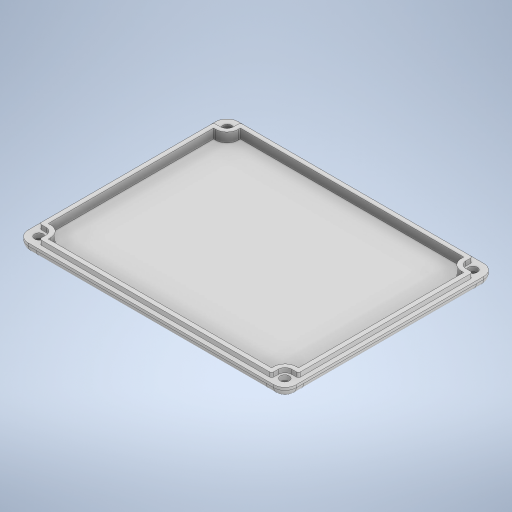
# Autodesk Inventor part: Couvercle_aluminium
Saved by Autodesk Inventor 2024 (Build 280153000, 153)
## iProperties
Created: 2024-08-30
Part Number: Couvercle_aluminium
Material: Générique
Document SubType Name: Modeling
Designer: malam
Density: 1 g/cm^3
Appearance: Par défaut
Author: malam
Autodesk Inventor part; units mm, degrees
ref_plane "YZ Plane" through (0, 0, 0) normal (1, 0, 0) x (0, 1, 0)
ref_plane "XZ Plane" through (0, 0, 0) normal (0, 1, 0) x (-1, 0, 0)
ref_plane "XY Plane" through (0, 0, 0) normal (0, 0, 1) x (1, 0, 0)
sketch "Esquisse1" plane through (0, 0, 0) normal (0, 1, 0) x (-1, 0, 0)
  arc A0 (55, -47) -> (60, -42) centre (55, -42) ccw
  line L0 (60, -42) -> (60, 42)
  arc A1 (60, 42) -> (55, 47) centre (55, 42) ccw
  line L1 (55, 47) -> (-55, 47)
  arc A2 (-55, 47) -> (-60, 42) centre (-55, 42) ccw
  line L2 (-60, 42) -> (-60, -42)
  arc A3 (-60, -42) -> (-55, -47) centre (-55, -42) ccw
  line L3 (-55, -47) -> (55, -47)
  circle A4 centre (55, 42.115) radius 2
  circle A5 centre (55, -42.115) radius 2
  circle A6 centre (-55, 42.115) radius 2
  circle A7 centre (-55, -42.115) radius 2
  arc A8 (55, -39) -> (52, -42) centre (55, -42) ccw
  line L4 (52, -42) -> (52, -44)
  arc A9 (51, -45) -> (52, -44) centre (51, -44) ccw
  line L5 (51, -45) -> (-51, -45)
  arc A10 (-52, -44) -> (-51, -45) centre (-51, -44) ccw
  line L6 (-52, -44) -> (-52, -42)
  arc A11 (-52, -42) -> (-55, -39) centre (-55, -42) ccw
  line L7 (-55, -39) -> (-57, -39)
  arc A12 (-58, -38) -> (-57, -39) centre (-57, -38) ccw
  line L8 (-58, -38) -> (-58, 38)
  arc A13 (-57, 39) -> (-58, 38) centre (-57, 38) ccw
  line L9 (-57, 39) -> (-55, 39)
  arc A14 (-55, 39) -> (-52, 42) centre (-55, 42) ccw
  line L10 (-52, 42) -> (-52, 44)
  arc A15 (-51, 45) -> (-52, 44) centre (-51, 44) ccw
  line L11 (-51, 45) -> (51, 45)
  arc A16 (52, 44) -> (51, 45) centre (51, 44) ccw
  line L12 (52, 44) -> (52, 42)
  arc A17 (52, 42) -> (55, 39) centre (55, 42) ccw
  line L13 (55, 39) -> (57, 39)
  arc A18 (58, 38) -> (57, 39) centre (57, 38) ccw
  line L14 (58, 38) -> (58, -38)
  arc A19 (57, -39) -> (58, -38) centre (57, -38) ccw
  line L15 (57, -39) -> (55, -39)
  line L16 (-50, -43) -> (50, -43)
  line L17 (50, -43) -> (50, -42)
  arc A20 (55, -37) -> (50, -42) centre (55, -42) ccw
  line L18 (55, -37) -> (56, -37)
  line L19 (56, -37) -> (56, 37)
  line L20 (56, 37) -> (55, 37)
  arc A21 (50, 42) -> (55, 37) centre (55, 42) ccw
  line L21 (50, 42) -> (50, 43)
  line L22 (50, 43) -> (-50, 43)
  line L23 (-50, 43) -> (-50, 42)
  arc A22 (-55, 37) -> (-50, 42) centre (-55, 42) ccw
  line L24 (-55, 37) -> (-56, 37)
  line L25 (-56, 37) -> (-56, -37)
  line L26 (-56, -37) -> (-55, -37)
  arc A23 (-50, -42) -> (-55, -37) centre (-55, -42) ccw
  line L27 (-50, -42) -> (-50, -43)
  point P0 (0, 0)
  point P1 (0, 0)
  dimension "d0" = 2
  constraints: 56 end point, 40 point on circle, 24 centre point, 15 other
  measures "d0" distance between parallel lines of L5 L16
extrude "Extrusion1" add sketch "Esquisse1" along normal blind 2 contours L27 A23 L26 L25 L24 A22 L23 L22 L21 A21 L20 L19 L18 A20 L17 L16
extrude "Extrusion2" add sketch "Esquisse1" along normal blind 6.2 contours A8 L4 A9 L5 A10 L6 A11 L7 A12 L8 A13 L9 A14 L10 A15 L11 A16 L12 A17 L13 A18 L14 A19 L15
extrude "Extrusion3" add sketch "Esquisse1" along normal blind 4.2 contours L3 A3 L2 A2 L1 A1 L0 A0
chamfer "Chanfrein1" distance 2 angle 45 4 edges at (57, 0, 42.115) (57, 0, -42.115) (-53, 0, -42.115) (-53, 0, 42.115)
fillet "Congé1" radius 3 8 edges at (58.5355, 0, 45.5355) (60, 0, 0) (58.5355, 0, -45.5355) (0, 0, -47) (-58.5355, 0, -45.5355) (-60, 0, 0) (-58.5355, 0, 45.5355) (0, 0, 47)
